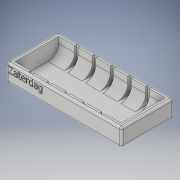
# Autodesk Inventor part: bakje woensdag
Saved by Autodesk Inventor 2019 (Build 230136000, 136)
## iProperties
Created: 2020-10-20
Part Number: bakje woensdag
Material: Generic
Document SubType Name: Modeling
Designer: daanswinters
Density: 1 g/cm^3
Appearance: Default
Author: daanswinters
Autodesk Inventor part; units mm, degrees
ref_plane "YZ Plane" through (0, 0, 0) normal (1, 0, 0) x (0, 1, 0)
ref_plane "XZ Plane" through (0, 0, 0) normal (0, 1, 0) x (-1, 0, 0)
ref_plane "XY Plane" through (0, 0, 0) normal (0, 0, 1) x (1, 0, 0)
sketch "Sketch1" plane through (0, 0, 0) normal (0, 0, 1) x (1, 0, 0)
  line L0 (55, -8.5) -> (-55, -8.5)
  line L1 (-55, -8.5) -> (-55, 8.5)
  line L2 (-55, 8.5) -> (55, 8.5)
  line L3 (55, 8.5) -> (55, -8.5)
  line L4 (55, -8.5) -> (-55, 8.5) construction
  line L5 (-55, -8.5) -> (55, 8.5) construction
  point P0 (0, 0)
  dimension "d0" = 110
  dimension "d1" = 17
  constraints: 12 end point, 2 midpoint, 2 parallel, 1 horizontal, 1 perpendicular
  measures "d0" distance of L1.end L2.end
  measures "d1" distance of L0.end L1.end
extrude "Extrusion1" add sketch "Sketch1" along normal blind 50
sketch "Sketch2" plane through (-55, 8.5, 0) normal (0, 1, 0) x (1, 0, 0)
  line L0 (0, 0) -> (0, -50) projected
  line L1 (110, -50) -> (0, -50)
  line L2 (0, -50) -> (0, 0)
  line L3 (0, 0) -> (110, 0)
  line L4 (110, 0) -> (110, -50)
  line L5 (110, -50) -> (0, 0) construction
  line L6 (0, -50) -> (110, 0) construction
  line L7 (106, -46) -> (106, -4)
  line L8 (4, -4) -> (4, -46)
  line L9 (56.15, -2) -> (53.85, -2)
  line L10 (53.85, -48) -> (56.15, -48)
  line L11 (56.15, -2) -> (53.85, -48) construction
  line L12 (53.85, -2) -> (56.15, -48) construction
  line L13 (73.15, -2) -> (70.85, -2)
  line L14 (70.85, -48) -> (73.15, -48)
  line L15 (73.15, -2) -> (70.85, -48) construction
  line L16 (70.85, -2) -> (73.15, -48) construction
  line L17 (0, -25) -> (110, -25) construction
  line L18 (87.85, -2) -> (90.15, -2)
  line L19 (90.15, -48) -> (87.85, -48)
  line L20 (87.85, -2) -> (90.15, -48) construction
  line L21 (90.15, -2) -> (87.85, -48) construction
  line L22 (36.85, -2) -> (39.15, -2)
  line L23 (39.15, -48) -> (36.85, -48)
  line L24 (36.85, -2) -> (39.15, -48) construction
  line L25 (39.15, -2) -> (36.85, -48) construction
  line L26 (19.85, -2) -> (22.15, -2)
  line L27 (22.15, -48) -> (19.85, -48)
  line L28 (19.85, -2) -> (22.15, -48) construction
  line L29 (22.15, -2) -> (19.85, -48) construction
  line L30 (90.15, -2) -> (90.15, -4)
  line L31 (90.15, -46) -> (90.15, -48)
  line L32 (87.85, -48) -> (87.85, -46)
  line L33 (87.85, -4) -> (87.85, -2)
  line L34 (73.15, -48) -> (73.15, -46)
  line L35 (73.15, -4) -> (73.15, -2)
  line L36 (70.85, -2) -> (70.85, -4)
  line L37 (70.85, -46) -> (70.85, -48)
  line L38 (56.15, -4) -> (56.15, -2)
  line L39 (53.85, -2) -> (53.85, -4)
  line L40 (53.85, -46) -> (53.85, -48)
  line L41 (56.15, -48) -> (56.15, -46)
  line L42 (39.15, -2) -> (39.15, -4)
  line L43 (39.15, -46) -> (39.15, -48)
  line L44 (36.85, -48) -> (36.85, -46)
  line L45 (36.85, -4) -> (36.85, -2)
  line L46 (22.15, -2) -> (22.15, -4)
  line L47 (19.85, -48) -> (19.85, -46)
  line L48 (19.85, -4) -> (19.85, -2)
  line L49 (22.15, -46) -> (22.15, -48)
  line L50 (4, -46) -> (19.95, -46)
  line L51 (22.05, -46) -> (36.95, -46)
  line L52 (39.05, -46) -> (53.95, -46)
  line L53 (56.05, -46) -> (70.95, -46)
  line L54 (73.05, -46) -> (87.95, -46)
  line L55 (90.05, -46) -> (106, -46)
  line L56 (106, -4) -> (90.05, -4)
  line L57 (87.95, -4) -> (73.05, -4)
  line L58 (70.95, -4) -> (56.05, -4)
  line L59 (53.95, -4) -> (39.05, -4)
  line L60 (36.95, -4) -> (22.05, -4)
  line L61 (19.95, -4) -> (4, -4)
  point P0 (55, 0)
  point P1 (55, -25)
  point P2 (72, -25)
  point P3 (89, -25)
  point P4 (38, -25)
  point P5 (21, -25)
  dimension "d4" = 65.556
  dimension "d5" = 110
  dimension "d7" = 2.3
  dimension "d8" = 46
  dimension "d9" = 2.3
  dimension "d10" = 46
  dimension "d11" = 0
  dimension "d12" = 2.3
  dimension "d13" = 46
  dimension "d14" = 2.3
  dimension "d15" = 46
  dimension "d16" = 2.3
  dimension "d17" = 46
  dimension "d18" = 17
  dimension "d19" = 17
  dimension "d20" = 17
  dimension "d21" = 17
  dimension "d22" = 2.862
  dimension "d23" = 2.862
  dimension "d24" = 106
  dimension "d25" = 4
  dimension "d26" = 42
  dimension "d27" = 2
  dimension "d28" = 0
  dimension "d29" = 42
  dimension "d30" = 0
  dimension "d31" = 42
  dimension "d32" = 0
  dimension "d33" = 42
  dimension "d34" = 0
  dimension "d35" = 42
  dimension "d36" = 0
  dimension "d37" = 42
  constraints: 122 end point, 73 parallel, 43 point on line, 17 perpendicular, 14 midpoint, 6 horizontal
  measures "d4" angle of L5 L0
  measures "d5" distance between parallel lines of L4 L0
  measures "d7" distance of L10.end L10.start
  measures "d8" distance of L10.start L9.end
  measures "d9" distance of L14.end L14.start
  measures "d10" distance of L14.start L13.end
  measures "d11" distance from line of L17 point (72, -25)
  measures "d12" distance of L19.start L19.end
  measures "d13" distance of L18.end L19.start
  measures "d14" distance of L23.start L23.end
  measures "d15" distance of L22.end L23.start
  measures "d16" distance of L27.start L27.end
  measures "d17" distance of L26.end L27.start
  measures "d18" distance of point (72, -25) point (55, -25)
  measures "d19" distance of point (89, -25) point (72, -25)
  measures "d20" distance of point (38, -25) point (55, -25)
  measures "d21" distance of point (21, -25) point (38, -25)
  measures "d22" angle of L0 L20
  measures "d23" angle of L0 L21
  measures "d24" distance between parallel lines of L7 L0
  measures "d25" distance between parallel lines of L8 L0
  measures "d26" distance between parallel lines of L56 L55
  measures "d27" distance between parallel lines of L56 L18
  measures "d28" distance between parallel lines of L56 L57
  measures "d29" distance between parallel lines of L56 L54
  measures "d30" distance between parallel lines of L56 L58
  measures "d31" distance between parallel lines of L56 L53
  measures "d32" distance between parallel lines of L56 L59
  measures "d33" distance between parallel lines of L56 L52
  measures "d34" distance between parallel lines of L56 L60
  measures "d35" distance between parallel lines of L56 L51
  measures "d36" distance between parallel lines of L56 L61
  measures "d37" distance between parallel lines of L56 L50
extrude "Extrusion2" cut sketch "Sketch2" against normal blind 16 contours L55 L31 L19 L32 L54 L34 L14 L37 L53 L41 L10 L40 L52 L43 L23 L44 L51 L49 L27 L47 L50 L8 L61 L48 L26 L46 L60 L45 L22 L42 L59 L39 L9 L38 L58 L36 L13 L35 L57 L33 L18 L30 L56 L7
fillet "Fillet1" radius 2 12 edges at (-55, 0, 50) (-55, 0, 0) (55, 0, 50) (55, 0, 0) (0, 8.5, 50) (-55, 8.5, 25) (0, 8.5, 0) (55, 8.5, 25) (55, -8.5, 25) (0, -8.5, 50) (-55, -8.5, 25) (0, -8.5, 0)
fillet "Fillet2" radius 10 6 edges at (-43.075, -7.5, 4) (-25.5, -7.5, 4) (-8.5, -7.5, 4) (8.5, -7.5, 4) (25.5, -7.5, 4) (43.075, -7.5, 4)
sketch "Sketch3" plane through (35.15, 8.5, 4) normal (0, 1, 0) x (1, 0, 0)
  line L0 (-70.3, -44) -> (-70.3, -42) projected
  line L1 (-51, 2) -> (-53.3, 2)
  line L2 (-34, 2) -> (-34, 0) projected
  line L3 (-36.3, -44) -> (-36.3, -42) projected
  line L4 (-19.3, -44) -> (-19.3, -42) projected
  line L5 (-2.3, -44) -> (-2.3, -42) projected
  line L6 (0, 2) -> (0, 0) projected
  line L7 (-19.8, 2) -> (-16.5, 2)
  line L8 (-16.5, 2) -> (-16.5, -44)
  line L9 (-16.5, -44) -> (-19.8, -44)
  line L10 (-19.8, -44) -> (-19.8, 2)
  line L11 (-19.8, 2) -> (-16.5, -44) construction
  line L12 (-16.5, 2) -> (-19.8, -44) construction
  line L13 (-2.8, -44) -> (0.5, -44)
  line L14 (0.5, -44) -> (0.5, 2)
  line L15 (0.5, 2) -> (-2.8, 2)
  line L16 (-2.8, 2) -> (-2.8, -44)
  line L17 (-2.8, -44) -> (0.5, 2) construction
  line L18 (0.5, -44) -> (-2.8, 2) construction
  line L19 (-36.8, -44) -> (-33.5, -44)
  line L20 (-33.5, -44) -> (-33.5, 2)
  line L21 (-33.5, 2) -> (-36.8, 2)
  line L22 (-36.8, 2) -> (-36.8, -44)
  line L23 (-36.8, -44) -> (-33.5, 2) construction
  line L24 (-33.5, -44) -> (-36.8, 2) construction
  line L25 (-51, 2) -> (-36.3, 2) projected
  line L26 (-53.8, -44) -> (-50.5, -44)
  line L27 (-50.5, -44) -> (-50.5, 2)
  line L28 (-50.5, 2) -> (-53.8, 2)
  line L29 (-53.8, 2) -> (-53.8, -44)
  line L30 (-53.8, -44) -> (-50.5, 2) construction
  line L31 (-50.5, -44) -> (-53.8, 2) construction
  line L32 (-53.3, -44) -> (-68, -44) projected
  line L33 (-70.8, 2) -> (-67.5, 2)
  line L34 (-67.5, 2) -> (-67.5, -44)
  line L35 (-67.5, -44) -> (-70.8, -44)
  line L36 (-70.8, -44) -> (-70.8, 2)
  line L37 (-70.8, 2) -> (-67.5, -44) construction
  line L38 (-67.5, 2) -> (-70.8, -44) construction
  point P0 (-35.15, 4)
  point P1 (-68, 2)
  point P2 (-17, 2)
  point P3 (-18.15, -21)
  point P4 (-1.15, -21)
  point P5 (-35.15, -21)
  point P6 (-52.15, -21)
  point P7 (-69.15, -21)
  dimension "d42" = 3.3
  dimension "d43" = 46
  dimension "d44" = 3.3
  dimension "d45" = 3.3
  dimension "d46" = 3.3
  dimension "d47" = 3.3
  dimension "d48" = 90
  dimension "d49" = 0.5
  dimension "d50" = 16.5
  dimension "d51" = 33.5
  dimension "d52" = 50.5
  dimension "d53" = 67.5
  dimension "d54" = 46
  dimension "d55" = 0
  dimension "d56" = 53.3
  constraints: 62 end point, 14 parallel, 10 midpoint, 5 horizontal, 5 perpendicular, 3 point on line
  measures "d42" distance of L8.end L9.end
  measures "d43" distance of L7.end L8.end
  measures "d44" distance of L15.end L14.end
  measures "d45" distance of L21.end L20.end
  measures "d46" distance of L28.end L27.end
  measures "d47" distance of L34.end L35.end
  measures "d48" angle of L6 L1
  measures "d49" distance between parallel lines of L6 L14
  measures "d50" distance between parallel lines of L6 L8
  measures "d51" distance between parallel lines of L6 L20
  measures "d52" distance between parallel lines of L6 L27
  measures "d53" distance between parallel lines of L6 L34
  measures "d54" distance between parallel lines of L25 L9
  measures "d55" distance between parallel lines of L15 L25
  measures "d56" distance from line of L1.end L6
extrude "Extrusion3" cut sketch "Sketch3" against normal blind 16
sketch "Sketch4" plane through (0, 0, 50) normal (0, 0, 1) x (1, 0, 0)
  line L0 (-52.9749, 6.5012) -> (53.0345, 6.5012) construction
  line L1 (53.0345, 6.5012) -> (53.0345, -6.5247) construction
  line L2 (53.0345, -6.5247) -> (-52.9749, -6.5247) construction
  line L3 (-52.9749, -6.5247) -> (-52.9749, 6.5012) construction
  line L4 (-48.4667, 0.1294) -> (-52.7278, 0.1294)
  line L5 (-52.7278, 0.1294) -> (-52.7278, 0.8857)
  line L6 (-52.7278, 0.8857) -> (-49.4652, 5.5077)
  line L7 (-49.4652, 5.5077) -> (-52.5795, 5.5077)
  line L8 (-52.5795, 5.5077) -> (-52.5795, 6.2294)
  line L9 (-52.5795, 6.2294) -> (-48.5507, 6.2294)
  line L10 (-48.5507, 6.2294) -> (-48.5507, 5.4978)
  line L11 (-48.5507, 5.4978) -> (-51.8479, 0.8511)
  line L12 (-51.8479, 0.8511) -> (-48.4667, 0.8511)
  line L13 (-48.4667, 0.8511) -> (-48.4667, 0.1294)
  spline S0 degree 2 poles (-45.1744, 0.6138) (-45.2684, 0.5446) (-45.5847, 0.2974) (-45.733, 0.2233) knots 0 0 0 1 2 2 2
  spline S1 degree 2 poles (-45.733, 0.2233) (-45.9357, 0.1145) (-46.3163, 0.0008) (-46.6624, 0.0008) knots 0 0 0 1 2 2 2
  spline S2 degree 2 poles (-46.6624, 0.0008) (-46.9441, 0.0008) (-47.4533, 0.2134) (-47.6461, 0.4062) knots 0 0 0 1 2 2 2
  spline S3 degree 2 poles (-47.6461, 0.4062) (-47.829, 0.594) (-48.0514, 1.1477) (-48.0514, 1.4542) knots 0 0 0 1 2 2 2
  spline S4 degree 2 poles (-48.0514, 1.4542) (-48.0514, 1.9287) (-47.651, 2.601) (-47.216, 2.7938) knots 0 0 0 1 2 2 2
  spline S5 degree 2 poles (-47.216, 2.7938) (-46.8304, 2.9718) (-45.7825, 3.1052) (-45.1744, 3.1398) knots 0 0 0 1 2 2 2
  line L14 (-45.1744, 3.1398) -> (-45.1744, 3.2881)
  spline S6 degree 2 poles (-45.1744, 3.2881) (-45.1744, 3.5551) (-45.3376, 3.8863) (-45.4859, 3.9802) knots 0 0 0 1 2 2 2
  spline S7 degree 2 poles (-45.4859, 3.9802) (-45.6342, 4.0741) (-46.0593, 4.1334) (-46.2867, 4.1334) knots 0 0 0 1 2 2 2
  spline S8 degree 2 poles (-46.2867, 4.1334) (-46.5536, 4.1334) (-47.2753, 3.9752) (-47.6362, 3.822) knots 0 0 0 1 2 2 2
  line L15 (-47.6362, 3.822) -> (-47.6807, 3.822)
  line L16 (-47.6807, 3.822) -> (-47.6807, 4.608)
  spline S9 degree 2 poles (-47.6807, 4.608) (-47.4681, 4.6673) (-46.6723, 4.8156) (-46.2817, 4.8156) knots 0 0 0 1 2 2 2
  spline S10 degree 2 poles (-46.2817, 4.8156) (-45.8072, 4.8156) (-45.1596, 4.6673) (-44.9026, 4.4745) knots 0 0 0 1 2 2 2
  spline S11 degree 2 poles (-44.9026, 4.4745) (-44.6505, 4.2867) (-44.4033, 3.6885) (-44.4033, 3.2585) knots 0 0 0 1 2 2 2
  line L17 (-44.4033, 3.2585) -> (-44.4033, 0.1294)
  line L18 (-44.4033, 0.1294) -> (-45.1744, 0.1294)
  line L19 (-45.1744, 0.1294) -> (-45.1744, 0.6138)
  line L20 (-45.1744, 1.2564) -> (-45.1744, 2.5269)
  spline S12 degree 2 poles (-45.1744, 2.5269) (-45.4513, 2.5021) (-46.2867, 2.4181) (-46.5487, 2.339) knots 0 0 0 1 2 2 2
  spline S13 degree 2 poles (-46.5487, 2.339) (-46.8552, 2.2451) (-47.2556, 1.8546) (-47.2556, 1.5085) knots 0 0 0 1 2 2 2
  spline S14 degree 2 poles (-47.2556, 1.5085) (-47.2556, 1.1131) (-46.8107, 0.7127) (-46.3855, 0.7127) knots 0 0 0 1 2 2 2
  spline S15 degree 2 poles (-46.3855, 0.7127) (-46.0247, 0.7127) (-45.4315, 1.0241) (-45.1744, 1.2564) knots 0 0 0 1 2 2 2
  spline S16 degree 2 poles (-41.9366, 0.0404) (-42.5644, 0.0404) (-43.2713, 0.7572) (-43.2713, 1.5333) knots 0 0 0 1 2 2 2
  line L21 (-43.2713, 1.5333) -> (-43.2713, 4.0692)
  line L22 (-43.2713, 4.0692) -> (-43.7903, 4.0692)
  line L23 (-43.7903, 4.0692) -> (-43.7903, 4.7068)
  line L24 (-43.7903, 4.7068) -> (-43.2713, 4.7068)
  line L25 (-43.2713, 4.7068) -> (-43.2713, 6.0218)
  line L26 (-43.2713, 6.0218) -> (-42.5001, 6.0218)
  line L27 (-42.5001, 6.0218) -> (-42.5001, 4.7068)
  line L28 (-42.5001, 4.7068) -> (-41.0814, 4.7068)
  line L29 (-41.0814, 4.7068) -> (-41.0814, 4.0692)
  line L30 (-41.0814, 4.0692) -> (-42.5001, 4.0692)
  line L31 (-42.5001, 4.0692) -> (-42.5001, 1.8892)
  spline S17 degree 2 poles (-42.5001, 1.8892) (-42.5001, 1.5431) (-42.4754, 1.1625) (-42.3914, 0.9994) knots 0 0 0 1 2 2 2
  spline S18 degree 2 poles (-42.3914, 0.9994) (-42.3222, 0.856) (-42.0107, 0.7127) (-41.7438, 0.7127) knots 0 0 0 1 2 2 2
  spline S19 degree 2 poles (-41.7438, 0.7127) (-41.556, 0.7127) (-41.205, 0.8264) (-41.1259, 0.861) knots 0 0 0 1 2 2 2
  line L32 (-41.1259, 0.861) -> (-41.0814, 0.861)
  line L33 (-41.0814, 0.861) -> (-41.0814, 0.1689)
  spline S20 degree 2 poles (-41.0814, 0.1689) (-41.2989, 0.1096) (-41.7438, 0.0404) (-41.9366, 0.0404) knots 0 0 0 1 2 2 2
  spline S21 degree 2 poles (-38.5257, 0.0256) (-39.6231, 0.0256) (-40.8293, 1.2564) (-40.8293, 2.3934) knots 0 0 0 1 2 2 2
  spline S22 degree 2 poles (-40.8293, 2.3934) (-40.8293, 3.5106) (-39.6577, 4.8354) (-38.7136, 4.8354) knots 0 0 0 1 2 2 2
  spline S23 degree 2 poles (-38.7136, 4.8354) (-38.2885, 4.8354) (-37.631, 4.5882) (-37.3888, 4.3262) knots 0 0 0 1 2 2 2
  spline S24 degree 2 poles (-37.3888, 4.3262) (-37.1416, 4.0642) (-36.8796, 3.3079) (-36.8796, 2.7592) knots 0 0 0 1 2 2 2
  line L34 (-36.8796, 2.7592) -> (-36.8796, 2.339)
  line L35 (-36.8796, 2.339) -> (-40.0483, 2.339)
  spline S25 degree 2 poles (-40.0483, 2.339) (-40.0483, 1.5431) (-39.2475, 0.6978) (-38.5356, 0.6978) knots 0 0 0 1 2 2 2
  spline S26 degree 2 poles (-38.5356, 0.6978) (-38.2835, 0.6978) (-37.7941, 0.8115) (-37.5964, 0.9005) knots 0 0 0 1 2 2 2
  spline S27 degree 2 poles (-37.5964, 0.9005) (-37.3888, 0.9994) (-37.1021, 1.1724) (-37.0082, 1.2515) knots 0 0 0 1 2 2 2
  line L36 (-37.0082, 1.2515) -> (-36.9637, 1.2515)
  line L37 (-36.9637, 1.2515) -> (-36.9637, 0.4111)
  spline S28 degree 2 poles (-36.9637, 0.4111) (-37.0971, 0.3568) (-37.5025, 0.1986) (-37.6607, 0.1541) knots 0 0 0 1 2 2 2
  spline S29 degree 2 poles (-37.6607, 0.1541) (-37.8831, 0.0898) (-38.2489, 0.0256) (-38.5257, 0.0256) knots 0 0 0 1 2 2 2
  spline S30 degree 2 poles (-37.631, 2.9273) (-37.6409, 3.2387) (-37.7694, 3.6935) (-37.893, 3.8467) knots 0 0 0 1 2 2 2
  spline S31 degree 2 poles (-37.893, 3.8467) (-38.0265, 4.0197) (-38.4466, 4.2026) (-38.7581, 4.2026) knots 0 0 0 1 2 2 2
  spline S32 degree 2 poles (-38.7581, 4.2026) (-39.0646, 4.2026) (-39.4946, 4.0197) (-39.6726, 3.8418) knots 0 0 0 1 2 2 2
  spline S33 degree 2 poles (-39.6726, 3.8418) (-39.8456, 3.6589) (-40.0235, 3.2189) (-40.0483, 2.9273) knots 0 0 0 1 2 2 2
  line L38 (-40.0483, 2.9273) -> (-37.631, 2.9273)
  line L39 (-33.6714, 3.8813) -> (-33.711, 3.8813)
  spline S34 degree 2 poles (-33.711, 3.8813) (-33.8, 3.906) (-33.9928, 3.9159) (-34.1262, 3.9159) knots 0 0 0 1 2 2 2
  spline S35 degree 2 poles (-34.1262, 3.9159) (-34.4376, 3.9159) (-35.0506, 3.644) (-35.3274, 3.3771) knots 0 0 0 1 2 2 2
  line L40 (-35.3274, 3.3771) -> (-35.3274, 0.1294)
  line L41 (-35.3274, 0.1294) -> (-36.0986, 0.1294)
  line L42 (-36.0986, 0.1294) -> (-36.0986, 4.7068)
  line L43 (-36.0986, 4.7068) -> (-35.3274, 4.7068)
  line L44 (-35.3274, 4.7068) -> (-35.3274, 4.0247)
  spline S36 degree 2 poles (-35.3274, 4.0247) (-34.9073, 4.4004) (-34.2795, 4.7068) (-33.9829, 4.7068) knots 0 0 0 1 2 2 2
  spline S37 degree 2 poles (-33.9829, 4.7068) (-33.8642, 4.7068) (-33.7456, 4.697) (-33.6714, 4.6821) knots 0 0 0 1 2 2 2
  line L45 (-33.6714, 4.6821) -> (-33.6714, 3.8813)
  line L46 (-29.5537, 0.1294) -> (-30.3248, 0.1294)
  line L47 (-30.3248, 0.1294) -> (-30.3248, 0.594)
  spline S38 degree 2 poles (-30.3248, 0.594) (-30.5028, 0.4457) (-30.7648, 0.248) (-30.9428, 0.164) knots 0 0 0 1 2 2 2
  spline S39 degree 2 poles (-30.9428, 0.164) (-31.1059, 0.0849) (-31.4569, 0.0008) (-31.6892, 0.0008) knots 0 0 0 1 2 2 2
  spline S40 degree 2 poles (-31.6892, 0.0008) (-32.0649, 0.0008) (-32.6976, 0.3123) (-32.9201, 0.6138) knots 0 0 0 1 2 2 2
  spline S41 degree 2 poles (-32.9201, 0.6138) (-33.1425, 0.9153) (-33.3897, 1.8051) (-33.3897, 2.3835) knots 0 0 0 1 2 2 2
  spline S42 degree 2 poles (-33.3897, 2.3835) (-33.3897, 2.9866) (-33.0782, 3.8665) (-32.8064, 4.1977) knots 0 0 0 1 2 2 2
  spline S43 degree 2 poles (-32.8064, 4.1977) (-32.5543, 4.4943) (-31.8474, 4.8354) (-31.4569, 4.8354) knots 0 0 0 1 2 2 2
  spline S44 degree 2 poles (-31.4569, 4.8354) (-31.1158, 4.8354) (-30.6066, 4.6821) (-30.3248, 4.5239) knots 0 0 0 1 2 2 2
  line L48 (-30.3248, 4.5239) -> (-30.3248, 6.5012)
  line L49 (-30.3248, 6.5012) -> (-29.5537, 6.5012)
  line L50 (-29.5537, 6.5012) -> (-29.5537, 0.1294)
  line L51 (-30.3248, 1.2416) -> (-30.3248, 3.8863)
  spline S45 degree 2 poles (-30.3248, 3.8863) (-30.6116, 4.0247) (-31.0663, 4.1285) (-31.3283, 4.1285) knots 0 0 0 1 2 2 2
  spline S46 degree 2 poles (-31.3283, 4.1285) (-31.9215, 4.1285) (-32.5938, 3.2387) (-32.5938, 2.3983) knots 0 0 0 1 2 2 2
  spline S47 degree 2 poles (-32.5938, 2.3983) (-32.5938, 1.5876) (-32.0797, 0.7324) (-31.5112, 0.7324) knots 0 0 0 1 2 2 2
  spline S48 degree 2 poles (-31.5112, 0.7324) (-31.2097, 0.7324) (-30.5967, 1.0093) (-30.3248, 1.2416) knots 0 0 0 1 2 2 2
  spline S49 degree 2 poles (-25.8858, 0.6138) (-25.9797, 0.5446) (-26.2961, 0.2974) (-26.4444, 0.2233) knots 0 0 0 1 2 2 2
  spline S50 degree 2 poles (-26.4444, 0.2233) (-26.647, 0.1145) (-27.0277, 0.0008) (-27.3737, 0.0008) knots 0 0 0 1 2 2 2
  spline S51 degree 2 poles (-27.3737, 0.0008) (-27.6555, 0.0008) (-28.1646, 0.2134) (-28.3574, 0.4062) knots 0 0 0 1 2 2 2
  spline S52 degree 2 poles (-28.3574, 0.4062) (-28.5403, 0.594) (-28.7628, 1.1477) (-28.7628, 1.4542) knots 0 0 0 1 2 2 2
  spline S53 degree 2 poles (-28.7628, 1.4542) (-28.7628, 1.9287) (-28.3624, 2.601) (-27.9274, 2.7938) knots 0 0 0 1 2 2 2
  spline S54 degree 2 poles (-27.9274, 2.7938) (-27.5418, 2.9718) (-26.4938, 3.1052) (-25.8858, 3.1398) knots 0 0 0 1 2 2 2
  line L52 (-25.8858, 3.1398) -> (-25.8858, 3.2881)
  spline S55 degree 2 poles (-25.8858, 3.2881) (-25.8858, 3.5551) (-26.0489, 3.8863) (-26.1972, 3.9802) knots 0 0 0 1 2 2 2
  spline S56 degree 2 poles (-26.1972, 3.9802) (-26.3455, 4.0741) (-26.7706, 4.1334) (-26.998, 4.1334) knots 0 0 0 1 2 2 2
  spline S57 degree 2 poles (-26.998, 4.1334) (-27.265, 4.1334) (-27.9867, 3.9752) (-28.3475, 3.822) knots 0 0 0 1 2 2 2
  line L53 (-28.3475, 3.822) -> (-28.392, 3.822)
  line L54 (-28.392, 3.822) -> (-28.392, 4.608)
  spline S58 degree 2 poles (-28.392, 4.608) (-28.1795, 4.6673) (-27.3836, 4.8156) (-26.9931, 4.8156) knots 0 0 0 1 2 2 2
  spline S59 degree 2 poles (-26.9931, 4.8156) (-26.5185, 4.8156) (-25.871, 4.6673) (-25.6139, 4.4745) knots 0 0 0 1 2 2 2
  spline S60 degree 2 poles (-25.6139, 4.4745) (-25.3618, 4.2867) (-25.1146, 3.6885) (-25.1146, 3.2585) knots 0 0 0 1 2 2 2
  line L55 (-25.1146, 3.2585) -> (-25.1146, 0.1294)
  line L56 (-25.1146, 0.1294) -> (-25.8858, 0.1294)
  line L57 (-25.8858, 0.1294) -> (-25.8858, 0.6138)
  line L58 (-25.8858, 1.2564) -> (-25.8858, 2.5269)
  spline S61 degree 2 poles (-25.8858, 2.5269) (-26.1626, 2.5021) (-26.998, 2.4181) (-27.26, 2.339) knots 0 0 0 1 2 2 2
  spline S62 degree 2 poles (-27.26, 2.339) (-27.5665, 2.2451) (-27.9669, 1.8546) (-27.9669, 1.5085) knots 0 0 0 1 2 2 2
  spline S63 degree 2 poles (-27.9669, 1.5085) (-27.9669, 1.1131) (-27.522, 0.7127) (-27.0969, 0.7127) knots 0 0 0 1 2 2 2
  spline S64 degree 2 poles (-27.0969, 0.7127) (-26.736, 0.7127) (-26.1428, 1.0241) (-25.8858, 1.2564) knots 0 0 0 1 2 2 2
  spline S65 degree 2 poles (-23.8689, -0.6022) (-23.7898, -0.6368) (-23.4883, -0.7456) (-23.2955, -0.7901) knots 0 0 0 1 2 2 2
  spline S66 degree 2 poles (-23.2955, -0.7901) (-23.0829, -0.8445) (-22.7221, -0.9087) (-22.5095, -0.9087) knots 0 0 0 1 2 2 2
  spline S67 degree 2 poles (-22.5095, -0.9087) (-22.1536, -0.9087) (-21.6593, -0.7209) (-21.5209, -0.5528) knots 0 0 0 1 2 2 2
  spline S68 degree 2 poles (-21.5209, -0.5528) (-21.3874, -0.3847) (-21.2836, 0.0552) (-21.2836, 0.337) knots 0 0 0 1 2 2 2
  line L59 (-21.2836, 0.337) -> (-21.2836, 0.7374)
  spline S69 degree 2 poles (-21.2836, 0.7374) (-21.595, 0.4655) (-22.1932, 0.2085) (-22.643, 0.2085) knots 0 0 0 1 2 2 2
  spline S70 degree 2 poles (-22.643, 0.2085) (-23.424, 0.2085) (-24.3484, 1.3701) (-24.3484, 2.4626) knots 0 0 0 1 2 2 2
  spline S71 degree 2 poles (-24.3484, 2.4626) (-24.3484, 3.0311) (-24.0271, 3.911) (-23.7602, 4.2224) knots 0 0 0 1 2 2 2
  spline S72 degree 2 poles (-23.7602, 4.2224) (-23.5031, 4.5141) (-22.7962, 4.8354) (-22.4205, 4.8354) knots 0 0 0 1 2 2 2
  spline S73 degree 2 poles (-22.4205, 4.8354) (-22.0646, 4.8354) (-21.5456, 4.6673) (-21.2836, 4.5141) knots 0 0 0 1 2 2 2
  line L60 (-21.2836, 4.5141) -> (-21.2391, 4.7068)
  line L61 (-21.2391, 4.7068) -> (-20.5124, 4.7068)
  line L62 (-20.5124, 4.7068) -> (-20.5124, 0.6534)
  spline S74 degree 2 poles (-20.5124, 0.6534) (-20.5124, -0.5133) (-21.5258, -1.6008) (-22.5688, -1.6008) knots 0 0 0 1 2 2 2
  spline S75 degree 2 poles (-22.5688, -1.6008) (-22.905, -1.6008) (-23.6069, -1.492) (-23.9085, -1.403) knots 0 0 0 1 2 2 2
  line L63 (-23.9085, -1.403) -> (-23.9085, -0.6022)
  line L64 (-23.9085, -0.6022) -> (-23.8689, -0.6022)
  line L65 (-21.2836, 1.3701) -> (-21.2836, 3.8863)
  spline S76 degree 2 poles (-21.2836, 3.8863) (-21.5703, 4.0247) (-22.0547, 4.1433) (-22.297, 4.1433) knots 0 0 0 1 2 2 2
  spline S77 degree 2 poles (-22.297, 4.1433) (-22.8803, 4.1433) (-23.5526, 3.2832) (-23.5526, 2.4774) knots 0 0 0 1 2 2 2
  spline S78 degree 2 poles (-23.5526, 2.4774) (-23.5526, 1.7162) (-23.0434, 0.9203) (-22.47, 0.9203) knots 0 0 0 1 2 2 2
  spline S79 degree 2 poles (-22.47, 0.9203) (-22.1684, 0.9203) (-21.5357, 1.1576) (-21.2836, 1.3701) knots 0 0 0 1 2 2 2
  point P0 (0, 0)
  constraints: 2 other
extrude "Extrusion4" cut sketch "Sketch4" against normal blind 0.5
fillet "Fillet3" radius 10 6 edges at (-43.325, -7.5, 46) (-25.5, -7.5, 46) (-8.5, -7.5, 46) (8.5, -7.5, 46) (25.5, -7.5, 46) (43.325, -7.5, 46)
body "Solid1"
